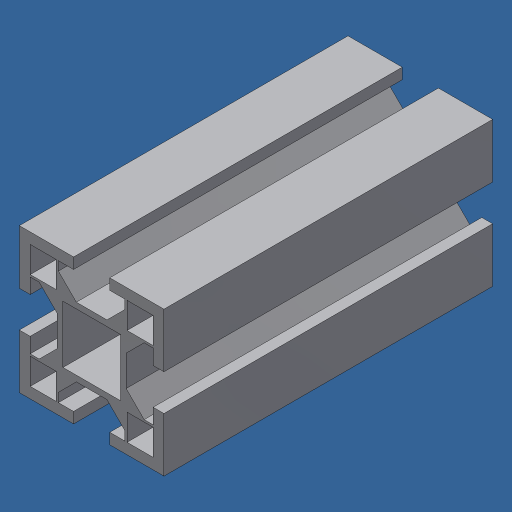
# Autodesk Inventor part: BAR, EXTRUDED, ALUM, 44MMX44MM, JOKAB
Saved by Autodesk Inventor 2024.3 (Build 283343000, 343)
## iProperties
ILogicPurgeVersion: 2.2.20.20
OnSaveVersion: 2.2.20.20
Category: _
Manager: _
Shininess: 64.0
Angle Display Precision: 2
Document Length Units: 11269
Document Angle Units: 11279
Document Time Units: 11290
Document Mass Units: 11283
Document Length Units Precision: 3
Document Angle Units Precision: 2
Part Number: BAR, EXTRUDED, ALUM, 44MMX44MM, JOKAB
Material: Aluminum, 6061
Document SubType Name: Modeling
Created: 2023-11-08
Designer: -
Manufacturer: Standard
Standards Organization: Custom
Density: 2.71 g/cm^3
Mass: 186.769 g
Surface Area: 527.015 cm^2
Volume: 68.9183 cm^3
Checked By: 00
Engr Approved By: R
User Status: Work In Process
Description: BAR, EXTRUDED, ALUM, 44MMX44MM, JOKAB
Mfg Approved By: Stephen.Oerton
Appearance: Aluminum - Flat
Density: 0.0
Volumn: 0.0
Area: 0.0
PropertySet Name: Model Information
Control State: 0
Master: False
Checked Out: False
CN_MASS: 0.19
CN_SERVICEABLE: _
CL_runCount: 0
FIRST_DESCRIPTION: _
SECOND_DESCRIPTION: _
THIRD_DESCRIPTION: _
ModelCat: Uncategorized
Author: -
Subject: _
Revision Number: A
Keywords: -
Autodesk Inventor part; units mm, degrees
ref_plane "YZ Plane" through (0, 0, 0) normal (1, 0, 0) x (0, 1, 0)
ref_plane "XZ Plane" through (0, 0, 0) normal (0, 1, 0) x (-1, 0, 0)
ref_plane "XY Plane" through (0, 0, 0) normal (0, 0, 1) x (1, 0, 0)
sketch "Sketch1" plane through (0, 0, 0) normal (0, 0, 1) x (1, 0, 0)
  line L0 (0, 0) -> (44, 0)
  line L1 (44, 0) -> (44, 44)
  line L2 (44, 44) -> (0, 44)
  line L3 (0, 44) -> (0, 0)
  dimension "d5" = 44
  dimension "d6" = 44
  constraints: 8 end point, 2 parallel, 1 horizontal, 1 perpendicular
  measures "d5" distance of L2.end L0.start
  measures "d6" distance of L0.start L0.end
extrude "JOKAB, 44MM" add sketch "Sketch1" along normal blind 100
sketch "Sketch2" plane through (0, 0, 100) normal (0, 0, 1) x (1, 0, 0)
  line L0 (44, 0) -> (0, 0) projected
  line L1 (0, 44) -> (44, 44) projected
  line L2 (44, 44) -> (0, 44) projected
  line L3 (16.5, 44) -> (16.5, 40.7)
  line L4 (11.875, 40.7) -> (11.875, 37.9667)
  line L5 (11.875, 37.9667) -> (17.3417, 32.5)
  line L6 (22, 44) -> (22, 0) construction
  line L7 (0, 44) -> (0, 0) projected
  line L8 (0, 22) -> (44, 22) construction
  line L9 (44, 0) -> (44, 44) projected
  line L10 (17.3417, 32.5) -> (22, 32.5)
  line L11 (11.875, 40.7) -> (16.5, 40.7)
  line L12 (27.5, 44) -> (27.5, 40.7)
  line L13 (32.125, 40.7) -> (32.125, 37.9667)
  line L14 (32.125, 37.9667) -> (26.6583, 32.5)
  line L15 (26.6583, 32.5) -> (22, 32.5)
  line L16 (32.125, 40.7) -> (27.5, 40.7)
  line L17 (16.5, 0) -> (16.5, 3.3)
  line L18 (11.875, 3.3) -> (11.875, 6.0333)
  line L19 (11.875, 6.0333) -> (17.3417, 11.5)
  line L20 (17.3417, 11.5) -> (22, 11.5)
  line L21 (11.875, 3.3) -> (16.5, 3.3)
  line L22 (27.5, 0) -> (27.5, 3.3)
  line L23 (32.125, 3.3) -> (27.5, 3.3)
  line L24 (32.125, 3.3) -> (32.125, 6.0333)
  line L25 (32.125, 6.0333) -> (26.6583, 11.5)
  line L26 (26.6583, 11.5) -> (22, 11.5)
  line L27 (0, 16.5) -> (3.3, 16.5)
  line L28 (3.3, 11.875) -> (6.0333, 11.875)
  line L29 (6.0333, 11.875) -> (11.5, 17.3417)
  line L30 (22, 0) -> (22, 44) construction
  line L31 (11.5, 17.3417) -> (11.5, 22)
  line L32 (3.3, 11.875) -> (3.3, 16.5)
  line L33 (0, 27.5) -> (3.3, 27.5)
  line L34 (3.3, 32.125) -> (3.3, 27.5)
  line L35 (3.3, 32.125) -> (6.0333, 32.125)
  line L36 (6.0333, 32.125) -> (11.5, 26.6583)
  line L37 (11.5, 26.6583) -> (11.5, 22)
  line L38 (27.5, 0) -> (27.5, 3.3)
  line L39 (32.125, 3.3) -> (32.125, 6.0333)
  line L40 (32.125, 6.0333) -> (26.6583, 11.5)
  line L41 (44, 22) -> (0, 22) construction
  line L42 (26.6583, 11.5) -> (22, 11.5)
  line L43 (32.125, 3.3) -> (27.5, 3.3)
  line L44 (16.5, 0) -> (16.5, 3.3)
  line L45 (11.875, 3.3) -> (16.5, 3.3)
  line L46 (11.875, 3.3) -> (11.875, 6.0333)
  line L47 (11.875, 6.0333) -> (17.3417, 11.5)
  line L48 (17.3417, 11.5) -> (22, 11.5)
  line L49 (44, 27.5) -> (40.7, 27.5)
  line L50 (40.7, 32.125) -> (37.9667, 32.125)
  line L51 (37.9667, 32.125) -> (32.5, 26.6583)
  line L52 (22, 44) -> (22, 0) construction
  line L53 (32.5, 26.6583) -> (32.5, 22)
  line L54 (40.7, 32.125) -> (40.7, 27.5)
  line L55 (44, 16.5) -> (40.7, 16.5)
  line L56 (40.7, 11.875) -> (40.7, 16.5)
  line L57 (40.7, 11.875) -> (37.9667, 11.875)
  line L58 (37.9667, 11.875) -> (32.5, 17.3417)
  line L59 (32.5, 17.3417) -> (32.5, 22)
  line L60 (27.5, 44) -> (16.5, 44)
  line L61 (44, 27.5) -> (44, 16.5)
  line L62 (27.5, 0) -> (16.5, 0)
  line L63 (0, 16.5) -> (0, 27.5)
  point P0 (22, 22)
  point P1 (22, 22)
  point P2 (22, 22)
  point P3 (22, 22)
  dimension "d10" = 5.5
  dimension "d11" = 10.125
  dimension "d12" = 11.5
  dimension "d13" = 45
  dimension "d15" = 2.7333
  dimension "d17" = 8.2
  dimension "d20" = 360
  constraints: 118 end point, 44 perpendicular, 16 symmetric about line, 5 midpoint, 4 coincident, 4 horizontal, 4 vertical, 2 point on line, 75 other
  measures "d10" distance between parallel lines of L6 L3
  measures "d11" distance between parallel lines of L6 L4
  measures "d12" distance between parallel lines of L1 L10
  measures "d13" angle of L10 L5
  measures "d15" distance of L4.start L4.end
  measures "d17" distance between parallel lines of L10 L11
extrude "Extrusion2" cut sketch "Sketch2" against normal through all contours L0 L17 L21 L18 L19 L20 L26 L25 L24 L23 L22 | L55 L56 L57 L58 L59 L53 L51 L50 L54 L49 L9 | L7 L33 L34 L35 L36 L37 L31 L29 L28 L32 L27 | L12 L16 L13 L14 L15 L10 L5 L4 L11 L3 L1
sketch "Sketch3" plane through (0, 0, 100) normal (0, 0, 1) x (1, 0, 0)
  line L0 (11.5, 26.6583) -> (11.5, 17.3417) projected
  line L1 (17.3417, 11.5) -> (26.6583, 11.5) projected
  line L2 (32.5, 17.3417) -> (32.5, 26.6583) projected
  line L3 (26.6583, 32.5) -> (17.3417, 32.5) projected
  line L4 (13.2688, 13.2687) -> (13.2687, 30.7313)
  line L5 (13.2687, 30.7313) -> (30.7312, 30.7313)
  line L6 (30.7312, 30.7313) -> (30.7313, 13.2688)
  line L7 (30.7313, 13.2688) -> (13.2688, 13.2687)
  line L8 (32.5, 22) -> (11.5, 22) construction
  line L9 (22, 32.5) -> (22, 11.5) construction
  dimension "d36" = 17.4625
  dimension "d37" = 8.7312
  dimension "d38" = 17.4625
  dimension "d39" = 8.7312
  constraints: 12 end point, 4 midpoint, 2 parallel, 1 perpendicular
  measures "d36" distance of L4.end L5.end
  measures "d37" distance between parallel lines of L6 L9
  measures "d38" distance of L5.end L6.end
  measures "d39" distance between parallel lines of L7 L8
extrude "Extrusion3" cut sketch "Sketch3" against normal through all
sketch "Sketch4" plane through (0, 0, 100) normal (0, 0, 1) x (1, 0, 0)
  line L0 (11.5, 26.6583) -> (11.5, 17.3417) projected
  line L1 (17.3417, 11.5) -> (26.6583, 11.5) projected
  line L2 (32.5, 17.3417) -> (32.5, 26.6583) projected
  line L3 (44, 44) -> (44, 27.5) projected
  line L4 (27.5, 44) -> (44, 44) projected
  line L5 (26.6583, 32.5) -> (17.3417, 32.5) projected
  line L6 (40.7, 32.7625) -> (32.7625, 32.7625)
  line L7 (32.7625, 32.7625) -> (32.7625, 40.7)
  line L8 (32.7625, 40.7) -> (40.7, 40.7)
  line L9 (40.7, 40.7) -> (40.7, 32.7625)
  line L10 (32.5, 22) -> (11.5, 22)
  line L11 (22, 32.5) -> (22, 11.5)
  line L12 (3.3, 32.7625) -> (11.2375, 32.7625)
  line L13 (11.2375, 32.7625) -> (11.2375, 40.7)
  line L14 (11.2375, 40.7) -> (3.3, 40.7)
  line L15 (3.3, 40.7) -> (3.3, 32.7625)
  line L16 (40.7, 11.2375) -> (32.7625, 11.2375)
  line L17 (32.7625, 11.2375) -> (32.7625, 3.3)
  line L18 (32.7625, 3.3) -> (40.7, 3.3)
  line L19 (40.7, 3.3) -> (40.7, 11.2375)
  line L20 (11.2375, 11.2375) -> (11.2375, 3.3)
  line L21 (11.2375, 3.3) -> (3.3, 3.3)
  line L22 (3.3, 3.3) -> (3.3, 11.2375)
  line L23 (3.3, 11.2375) -> (11.2375, 11.2375)
  dimension "d30" = 3.3
  dimension "d31" = 3.3
  dimension "d32" = 7.9375
  dimension "d33" = 7.9375
  constraints: 36 end point, 12 symmetric about line, 4 midpoint, 2 parallel, 1 horizontal, 1 perpendicular, 12 other
  measures "d30" distance between parallel lines of L4 L8
  measures "d31" distance between parallel lines of L3 L9
  measures "d32" distance of L6.end L7.end
  measures "d33" distance between parallel lines of L9 L7
extrude "Extrusion4" cut sketch "Sketch4" against normal through all
equation "\"d15\" = 0.333333 * d17"
equation "\"d37\" = 0.5 * d36"
equation "\"d38\" = d36"
equation "\"d39\" = d37"
equation "\"d31\" = d30"
equation "\"d33\" = d32"
